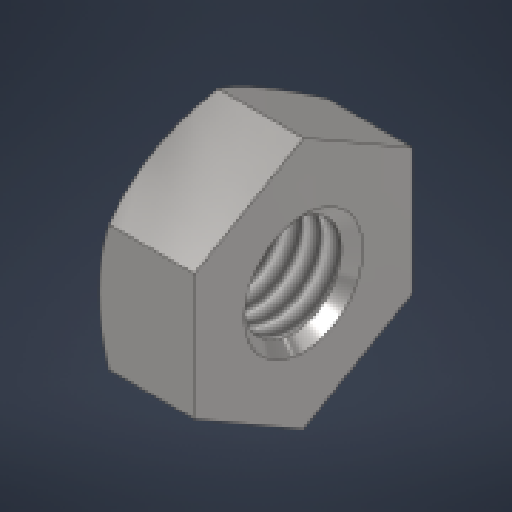
# Autodesk Inventor part: SLBNR3
Saved by Autodesk Inventor 2024 (Build 280153000, 153)
## iProperties
Created: 2023-10-29
Part Number: SLBNR3
Material: 스테인리스스틸
Catalog Web Link: www.cadenas.de
Description: LBNR, LBNL, SLBNR, SLBNL, KNTR, KNTL, SKNTR-Nuts
Vendor: MISUMI
Document SubType Name: Modeling
Designer: psAdmin
Manufacturer: MISUMI
Mass: 0.405507 g
Surface Area: 1.03677 cm^2
Volume: 0.0506884 cm^3
Density: 8 g/cm^3
Appearance: 반연마
Category: PARTsolutions
Company: MISUMI
PSOL_IDENT_0: {$CADENAS_DATA/23d-libs/misumi/metric/27_screws_nuts/slbnl.prj},199 {VTYP=3D},{NB=SLBNR3},{LINA=SLBN
PSOL_IDENT_1: R3},{NN=LBNR, LBNL, SLBNR, SLBNL, KNTR, KNTL, SKNTR},{DATE=03.06.2021 03:35:45},{GEOMDATE=05.11.2010
PSOL_IDENT_2: 00:00:00},{VERSION=},{LINEID=20},{WBVAR=TRS,MAT,CS},{WBNUMERIC=}  {NB=SLBNR3},{LINA=SLBNR3},{KT=DUM
PSOL_IDENT_3: MY},{PN=SLBNR3},{TS=LBN},{TRS=R},{MAT=S},{ST=-},{CS=1},{M1=3},{M=3.0},{P=0.50},{B=5.5},{EE=6.4},{T=2
PSOL_IDENT_4: .4},{T1=0.0},{TFX=2.4},{T1FX=1.8},{CALG='1','JIS Class 1','2','JIS Class 3'},{TRSALG= 'R', 'Right-Ha
PSOL_IDENT_5: nd Thread', 'L', 'Left-Hand Thread' },{MATALG= '', 'SWCH Carbon Steel', 'S', '304 Stainless Steel' }
NB: SLBNR3
NN: LBNR, LBNL, SLBNR, SLBNL, KNTR, KNTL, SKNTR
NT: Nuts
NBSYN: $PN.
LINA: SLBNR3
CATALOG: Misumi
PN: SLBNR3
TRS: Right-Hand Thread
MAT: 304 Stainless Steel Equivalent
ST: -
CS: JIS Class 1
M1: 3
P: 0.5
B: 5.5
EE: 6.4
T: 2.4
T1: 0
SUPPLIER: MISUMI
ARTICLENO: SLBNR3
BOMINFO: SLBNR3
CREATOR: CADENAS GmbH
Title: SLBNR3
Author: Cadenas PARTsolutions
Comments: Nuts
Autodesk Inventor part; units mm, degrees
sketch "Sketch_1" plane through (0, 0, 0) normal (0, 0, 1) x (1, 0, 0)
  line L0 (1.2, 0) -> (-1.2, 0)
  line L1 (-1.2, 0) -> (-1.2, 2.75)
  line L2 (-1.2, 2.75) -> (-0.9402, 3.2)
  line L3 (-0.9402, 3.2) -> (1.2, 3.2)
  line L4 (1.2, 3.2) -> (1.2, 0)
  line L5 (1.2, 0) -> (-1.2, 0)
  constraints: 12 end point
revolve "Revolution1" add sketch "Sketch_1" angle 360 about axis through (1.2, 0, 0) along (1, 0, 0)
sketch "Sketch_2" plane through (0, 0, 0) normal (0, 0, 1) x (1, 0, 0)
  line L0 (1.2, 0) -> (-1.2, 0)
  line L1 (-1.2, 0) -> (-1.2, 1.5)
  line L2 (-1.2, 1.5) -> (-0.9295, 1.2295)
  line L3 (-0.9295, 1.2295) -> (0.9295, 1.2295)
  line L4 (0.9295, 1.2295) -> (1.2, 1.5)
  line L5 (1.2, 1.5) -> (1.2, 0)
  line L6 (1.2, 0) -> (-1.2, 0)
  constraints: 14 end point
revolve "Revolution2" cut sketch "Sketch_2" angle 360 about axis through (1.2, 0, 0) along (1, 0, 0)
thread "Thread1" size "M3x0.5" class "6H" standard "ISO Metric profile" full length
sketch "Sketch_3" plane through (0, 0, 0) normal (1, 0, 0) x (0, 1, 0)
  line L0 (-5.5, 5.5) -> (-5.5, -5.5)
  line L1 (-5.5, -5.5) -> (5.5, -5.5)
  line L2 (5.5, -5.5) -> (5.5, 5.5)
  line L3 (5.5, 5.5) -> (-5.5, 5.5)
  line L4 (-1.5877, 2.75) -> (-3.1754, 0)
  line L5 (-3.1754, 0) -> (-1.5877, -2.75)
  line L6 (-1.5877, -2.75) -> (1.5877, -2.75)
  line L7 (1.5877, -2.75) -> (3.1754, 0)
  line L8 (3.1754, 0) -> (1.5877, 2.75)
  line L9 (1.5877, 2.75) -> (-1.5877, 2.75)
  constraints: 20 end point
extrude "Extrusion1" cut sketch "Sketch_3" along normal mid plane 2.4
ref_plane "cp_XY" through (1.2, 0, 0) normal (1, 0, 0) x (0, 0, -1)
ref_plane "cp_YZ" through (1.2, 0, 0) normal (0, 0, -1) x (0, 1, 0)
ref_plane "cp_ZX" through (1.2, 0, 0) normal (0, 1, 0) x (1, 0, 0)
ref_plane "nut_to_screw_XY" through (0, 0, 0) normal (1, 0, 0) x (0, 0, -1)
ref_plane "nut_to_screw_YZ" through (0, 0, 0) normal (0, 0, -1) x (0, 1, 0)
ref_plane "nut_to_screw_ZX" through (0, 0, 0) normal (0, 1, 0) x (1, 0, 0)
body "Solid1"
